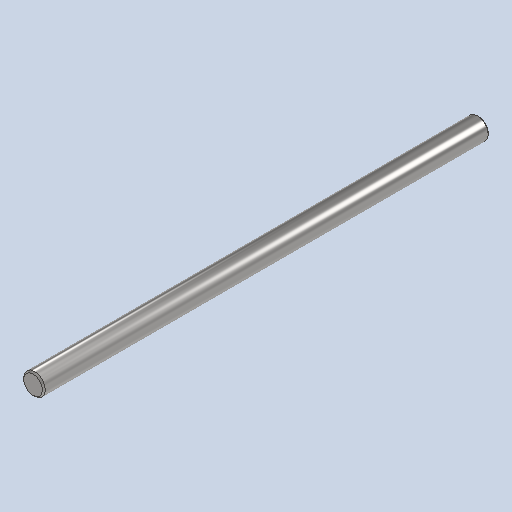
# Autodesk Inventor part: Shaft_6mmx62mm
Saved by Autodesk Inventor 2024 (Build 280153000, 153)
## iProperties
Created: 2022-09-14
Part Number: Shaft_6mmx62mm
Material: Edelstahl
Document SubType Name: Modeling
Designer: alexw
Density: 8 g/cm^3
Appearance: Halbpoliert
Mass: 3.50314 g
Surface Area: 5.96161 cm^2
Volume: 0.437892 cm^3
Author: alexw
Autodesk Inventor part; units mm, degrees
ref_plane "YZ Plane" through (0, 0, 0) normal (1, 0, 0) x (0, 1, 0)
ref_plane "XZ Plane" through (0, 0, 0) normal (0, 1, 0) x (-1, 0, 0)
ref_plane "XY Plane" through (0, 0, 0) normal (0, 0, 1) x (1, 0, 0)
sketch "Skizze1" plane through (0, 0, 0) normal (0, 0, 1) x (1, 0, 0)
  circle A0 centre (0, 0) radius 1.5
  dimension "d0" = 3
  constraints: 1 centre point, 1 coincident
  measures "d0" diameter of A0
extrude "Extrusion1" add sketch "Skizze1" along normal blind 62
chamfer "Fase1" distance 0.2 angle 45 2 edges at (-1.5, 0, 62) (-1.5, 0, 0)
